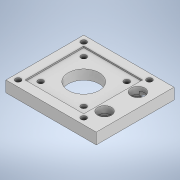
# Autodesk Inventor part: Linear Rail Front Plate
Saved by Autodesk Inventor 2022 (Build 260153000, 153)
## iProperties
Created: 2021-11-30
Part Number: Linear Rail Front Plate
Material: Generic
Document SubType Name: Modeling
Designer: efred
Density: 1 g/cm^3
Appearance: Default
Author: efred
Autodesk Inventor part; units mm, degrees
ref_plane "YZ Plane" through (0, 0, 0) normal (1, 0, 0) x (0, 1, 0)
ref_plane "XZ Plane" through (0, 0, 0) normal (0, 1, 0) x (-1, 0, 0)
ref_plane "XY Plane" through (0, 0, 0) normal (0, 0, 1) x (1, 0, 0)
sketch "Sketch1" plane through (0, 0, 0) normal (0, 1, 0) x (-1, 0, 0)
  line L0 (-32.5, 28) -> (32.5, 28)
  line L1 (32.5, 28) -> (32.5, -28)
  line L2 (32.5, -28) -> (-32.5, -28)
  line L3 (-32.5, -28) -> (-32.5, 28)
  line L4 (-32.5, 28) -> (32.5, -28) construction
  line L5 (32.5, 28) -> (-32.5, -28) construction
  circle A0 centre (4.5, 0) radius 11.15
  line L6 (-11, 15.5) -> (20, 15.5) construction
  line L7 (20, 15.5) -> (20, -15.5) construction
  line L8 (20, -15.5) -> (-11, -15.5) construction
  line L9 (-11, -15.5) -> (-11, 15.5) construction
  line L10 (-11, 15.5) -> (20, -15.5) construction
  line L11 (20, 15.5) -> (-11, -15.5) construction
  circle A1 centre (20, 15.5) radius 2
  line L12 (-11, 15.5) -> (20, 15.5) construction
  line L13 (20, 15.5) -> (20, -15.5) construction
  line L14 (20, -15.5) -> (-11, -15.5) construction
  line L15 (-11, -15.5) -> (-11, 15.5) construction
  circle A2 centre (-11, 15.5) radius 2
  line L16 (-11, -15.5) -> (-11, 15.5) construction
  line L17 (-11, 15.5) -> (20, 15.5) construction
  line L18 (20, 15.5) -> (20, -15.5) construction
  line L19 (20, -15.5) -> (-11, -15.5) construction
  circle A3 centre (-11, -15.5) radius 2
  line L20 (20, -15.5) -> (-11, -15.5) construction
  line L21 (-11, -15.5) -> (-11, 15.5) construction
  line L22 (-11, 15.5) -> (20, 15.5) construction
  line L23 (20, 15.5) -> (20, -15.5) construction
  circle A4 centre (20, -15.5) radius 2
  circle A5 centre (28.1317, 23.6317) radius 2
  line L24 (28.1317, 23.6317) -> (20, 15.5) construction
  circle A6 centre (-19.1317, 23.6317) radius 2
  circle A7 centre (-19.1317, -23.6317) radius 2
  circle A8 centre (28.1317, -23.6317) radius 2
  circle A9 centre (-22.5, -12) radius 3.15
  line L25 (32.5, 0) -> (-32.5, 0) construction
  circle A10 centre (-22.5, 12) radius 3.15
  point P0 (0, 0)
  point P1 (0, 0)
  dimension "d0" = 56
  dimension "d1" = 65
  dimension "d2" = 28
  dimension "d3" = 22.3
  dimension "d4" = 31
  dimension "d5" = 31
  dimension "d8" = 360
  dimension "d10" = 4
  dimension "d11" = 11.5
  dimension "d12" = 4
  dimension "d15" = 360
  dimension "d17" = 16
  dimension "d18" = 10
  dimension "d19" = 6.3
  constraints: 52 end point, 11 centre point, 7 midpoint, 4 coincident, 4 parallel, 2 horizontal, 2 perpendicular, 1 horizontal alignment, 1 point on line, 1 symmetric about line, 51 other
  measures "d0" distance between parallel lines of L2 L0
  measures "d1" distance between parallel lines of L3 L1
  measures "d2" distance from line of L1 A0.centre
  measures "d3" diameter of A0
  measures "d4" distance of L7.end L8.end
  measures "d5" distance of L6.end L7.end
  measures "d10" diameter of A1
  measures "d11" distance of L24.start L22.end
  measures "d12" diameter of A5
  measures "d17" distance from line of L2 A9.centre
  measures "d18" distance from line of L3 A9.centre
  measures "d19" diameter of A9
extrude "Extrusion1" add sketch "Sketch1" along normal blind 8
sketch "Sketch2" plane through (0, 8, 0) normal (0, 1, 0) x (1, 0, 0)
  circle A0 centre (-4.5, 0) radius 11.15 construction
  line L0 (16.65, -21.15) -> (-25.65, -21.15)
  line L1 (-25.65, -21.15) -> (-25.65, 21.15)
  line L2 (-25.65, 21.15) -> (16.65, 21.15)
  line L3 (16.65, 21.15) -> (16.65, -21.15)
  line L4 (16.65, -21.15) -> (-25.65, 21.15) construction
  line L5 (-25.65, -21.15) -> (16.65, 21.15) construction
  point P0 (0, 0)
  dimension "d22" = 42.3
  dimension "d23" = 42.3
  constraints: 12 end point, 2 midpoint, 2 parallel, 1 horizontal, 1 perpendicular
  measures "d22" distance of L1.end L2.end
  measures "d23" distance of L0.end L1.end
extrude "Extrusion2" cut sketch "Sketch2" against normal blind 1
sketch "Sketch3" plane through (0, 8, 0) normal (0, 1, 0) x (1, 0, 0)
  circle A0 centre (22.5, -12) radius 3.15 construction
  circle A1 centre (22.5, 12) radius 3.15 construction
  circle A2 centre (22.5, -12) radius 5
  circle A3 centre (22.5, 12) radius 5
  point P0 (0, 0)
  dimension "d26" = 10
  dimension "d27" = 10
  constraints: 2 centre point, 2 coincident
  measures "d26" diameter of A2
  measures "d27" diameter of A3
extrude "Extrusion3" cut sketch "Sketch3" against normal blind 5
sketch "Sketch4" plane through (0, 0, 0) normal (0, -1, 0) x (1, 0, 0)
  line L0 (32.5, -28) -> (-32.5, -28) projected
  line L1 (32.5, 28) -> (32.5, -28) projected
  line L2 (-32.5, 28) -> (32.5, 28) projected
  line L3 (-32.5, -28) -> (-32.5, 28) projected
  circle A0 centre (22.5, 12) radius 3.15 projected
  circle A1 centre (-28.1317, -23.6317) radius 2 projected
  circle A2 centre (-4.5, 0) radius 11.15 projected
  circle A3 centre (-20, 15.5) radius 2 projected
  circle A4 centre (11, 15.5) radius 2 projected
  circle A5 centre (11, -15.5) radius 2 projected
  circle A6 centre (-20, -15.5) radius 2 projected
  circle A7 centre (-28.1317, 23.6317) radius 2 projected
  circle A8 centre (19.1317, 23.6317) radius 2 projected
  circle A9 centre (19.1317, -23.6317) radius 2 projected
  circle A10 centre (22.5, -12) radius 3.15 projected
  circle A11 centre (-20, 15.5) radius 3
  circle A12 centre (-20, -15.5) radius 3
  circle A13 centre (11, -15.5) radius 3
  circle A14 centre (11, 15.5) radius 3
  circle A15 centre (21, 18.5) radius 3
  line L4 (-32.5, -28) -> (-32.5, 28) projected
  line L5 (-32.5, 0) -> (32.5, 0) construction
  circle A16 centre (21, -18.5) radius 3
  point P0 (0, 0)
  dimension "d30" = 6
  dimension "d33" = 360
  dimension "d35" = 9.5
  dimension "d36" = 11.5
  dimension "d37" = 6
  constraints: 6 centre point, 2 end point, 2 midpoint, 1 coincident, 1 symmetric about line, 10 other
  measures "d30" diameter of A11
  measures "d35" distance from line of L2 A15.centre
  measures "d36" distance from line of L1 A15.centre
  measures "d37" diameter of A15
extrude "Extrusion4" cut sketch "Sketch4" against normal blind 5 contours A3 | A4 | A5 | A6 | A11 | A12 | A13 | A14 | A15 | A16
body "Solid1"
